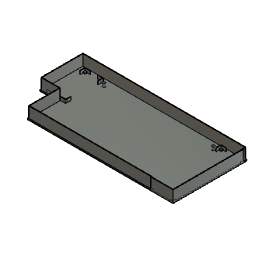
GeigerCounterBase v3 (Autodesk Fusion 360 design; units mm, degrees)
Autodesk Fusion 360 part; units mm, degrees
note: some values were not read from the file. Chosen so that the rebuilt part matches the saved one: which face or edge a step refers to; which pieces of a blend or face edit are solid.
(part 1 of 2)
sketch "Skizze1" plane through (0, 0, 0) normal (0, 1, 0) x (1, 0, 0)
  line L0 (0, 0) -> (133, 0)
  line L1 (133, 0) -> (133, -68.5)
  line L2 (133, -68.5) -> (0, -68.5)
  line L3 (0, -68.5) -> (0, 0)
  dimension "d1" = 133
  dimension "d2" = 68.5
  constraint horizontal L0
  constraint vertical L1
  constraint horizontal L2
  constraint vertical L3
  constraint coincident L0.start L3.end
  measures "d1" distance of L0.start L0.end
  measures "d2" distance of L0.start L2.end
extrude "Extrusion1" add sketch "Skizze1" along normal blind 1 makes body 1
sketch "Skizze2" plane through (0, 1, 0) normal (0, 1, 0) x (-1, 0, 0)
  line L0 (0, 68.5) -> (-133, 68.5)
  line L1 (-133, 68.5) -> (-133, 0)
  line L2 (-133, 0) -> (0, 0)
  line L3 (0, 0) -> (0, 68.5)
  circle A0 centre (-15, 10) radius 1.5
  dimension "d5" = 3
  measures "d5" diameter of A0
extrude "Extrusion2" add sketch "Skizze2" along normal blind 3 contours A0 bodies 1
pattern_linear "R-Anordnung1" count 2 spacing 10.15 along (1, 0, 0) of "Extrusion2"
delete_face "Fläche löschen1" 2 faces at (23.6519, 3, 9.9252) (25.4, 4, 10.4979) on bodies 1
delete_face "Fläche löschen2" 1 faces at (13.5019, 3, 9.9252) on bodies 1
sketch "Skizze3" plane through (0, 1, 0) normal (0, 1, 0) x (-1, 0, 0)
  line L0 (0, 68.5) -> (-133, 68.5)
  line L1 (-133, 68.5) -> (-133, 0)
  line L2 (-133, 0) -> (0, 0)
  line L3 (0, 0) -> (0, 68.5)
  circle A0 centre (-9.9603, 7.5483) radius 1.25
  dimension "d12" = 2.5
  measures "d12" diameter of A0
extrude "Extrusion3" add sketch "Skizze3" along normal blind 3 contours A0 bodies 1
pattern_linear "R-Anordnung2" count 2 spacing 101.5 along (1, 0, 0) of "Extrusion3"
pattern_linear "R-Anordnung3" count 2 spacing 56.5 along (0, 0, 1) of "Extrusion3"
pattern_linear "R-Anordnung4" count 2 spacing 101.5 along (1, 0, 0) of "R-Anordnung3"
sketch "Skizze4" plane through (0, 1, 0) normal (0, 1, 0) x (-1, 0, 0)
  circle A0 centre (-111.4603, 64.0483) radius 1.25
  circle A1 centre (-9.9603, 64.0483) radius 1.25
  circle A2 centre (-111.4603, 7.5483) radius 1.25
  circle A3 centre (-9.9603, 7.5483) radius 1.25
  line L0 (0, 68.5) -> (-133, 68.5)
  line L1 (-133, 68.5) -> (-133, 0)
  line L2 (-133, 0) -> (0, 0)
  line L3 (0, 0) -> (0, 68.5)
  line L4 (-133, 68.5) -> (-128, 68.5)
  line L5 (-128, 68.5) -> (-128, 68)
  line L6 (-128, 68) -> (-133, 68)
  line L7 (-133, 68) -> (-133, 68.5)
  dimension "d27" = 5
  constraint horizontal L4
  constraint vertical L5
  constraint horizontal L6
  constraint vertical L7
  constraint coincident L0.end L1.start
  measures "d27" distance of L0.end L4.end
extrude "Extrusion4" add sketch "Skizze4" along normal blind 3 contours L0 L1 L4 L5 L6 L7 bodies 1
sketch "Skizze5" plane through (0, 1, 0) normal (0, 1, 0) x (-1, 0, 0)
  line L0 (-128, 68.5) -> (-128, 68)
  line L1 (-128, 68) -> (-133, 68)
  line L2 (-133, 68) -> (-133, 0)
  line L3 (-133, 0) -> (0, 0)
  line L4 (0, 0) -> (0, 68.5)
  line L5 (0, 68.5) -> (-128, 68.5)
  circle A0 centre (-9.9603, 7.5483) radius 1.25
  circle A1 centre (-111.4603, 7.5483) radius 1.25
  circle A2 centre (-9.9603, 64.0483) radius 1.25
  circle A3 centre (-111.4603, 64.0483) radius 1.25
  line L6 (-133, 68) -> (-132.5, 68)
  line L7 (-132.5, 68) -> (-132.5, 63.5)
  line L8 (-132.5, 63.5) -> (-133, 63.5)
  line L9 (-133, 63.5) -> (-133, 68)
  dimension "d30" = 0.5
  dimension "d31" = 4.5
  constraint horizontal L6
  constraint vertical L7
  constraint horizontal L8
  constraint vertical L9
  constraint coincident L1.end L2.start
  measures "d30" distance of L1.end L6.end
  measures "d31" distance of L1.end L8.end
extrude "Extrusion5" add sketch "Skizze5" along normal blind 3 contours L1 L2 L6 L7 L8 L9 bodies 1
sketch "Skizze6" plane through (0, 1, 0) normal (0, 1, 0) x (-1, 0, 0)
  line L0 (-132.5, 63.5) -> (-133, 63.5)
  line L1 (-133, 63.5) -> (-133, 0)
  line L2 (-133, 0) -> (0, 0)
  line L3 (0, 0) -> (0, 68.5)
  line L4 (0, 68.5) -> (-128, 68.5)
  line L5 (-128, 68.5) -> (-128, 68)
  line L6 (-128, 68) -> (-132.5, 68)
  line L7 (-132.5, 68) -> (-132.5, 63.5)
  circle A0 centre (-9.9603, 7.5483) radius 1.25
  circle A1 centre (-111.4603, 7.5483) radius 1.25
  circle A2 centre (-9.9603, 64.0483) radius 1.25
  circle A3 centre (-111.4603, 64.0483) radius 1.25
  line L8 (-132.5, 68) -> (-130.5, 68)
  line L9 (-130.5, 68) -> (-130.5, 66)
  line L10 (-130.5, 66) -> (-132.5, 66)
  line L11 (-132.5, 66) -> (-132.5, 68)
  dimension "d34" = 2
  dimension "d35" = 2
  constraint horizontal L8
  constraint vertical L9
  constraint horizontal L10
  constraint vertical L11
  constraint coincident L6.end L7.start
  measures "d34" distance of L6.end L8.end
  measures "d35" distance of L6.end L10.end
extrude "Extrusion6" add sketch "Skizze6" along normal blind 1 contours L6 L7 L8 L9 L10 L11 bodies 1
sketch "Skizze7" plane through (0, 1, 0) normal (0, 1, 0) x (-1, 0, 0)
  line L0 (-130.5, 66) -> (-132.5, 66)
  line L1 (-132.5, 66) -> (-132.5, 63.5)
  line L2 (-132.5, 63.5) -> (-133, 63.5)
  line L3 (-133, 63.5) -> (-133, 0)
  line L4 (-133, 0) -> (0, 0)
  line L5 (0, 0) -> (0, 68.5)
  line L6 (0, 68.5) -> (-128, 68.5)
  line L7 (-128, 68.5) -> (-128, 68)
  line L8 (-128, 68) -> (-130.5, 68)
  line L9 (-130.5, 68) -> (-130.5, 66)
  circle A0 centre (-9.9603, 7.5483) radius 1.25
  circle A1 centre (-111.4603, 7.5483) radius 1.25
  circle A2 centre (-9.9603, 64.0483) radius 1.25
  circle A3 centre (-111.4603, 64.0483) radius 1.25
  line L10 (-135, 0) -> (-133, 0)
  line L11 (-133, 0) -> (-133, 68.5)
  line L12 (-133, 68.5) -> (-135, 68.5)
  line L13 (-135, 68.5) -> (-135, 0)
  dimension "d38" = 68.5
  constraint horizontal L10
  constraint vertical L11
  constraint horizontal L12
  constraint vertical L13
  measures "d38" distance of L10.start L12.end
extrude "Extrusion7" add sketch "Skizze7" against normal blind 1 contours L3 L10 L11 L12 L13 bodies 1
delete_face "Fläche löschen3" 1 faces at (133, 2, 66.8333) on bodies 1
sketch "Skizze8" plane through (0, 1, 0) normal (0, 1, 0) x (-1, 0, 0)
  circle A0 centre (-9.9603, 7.5483) radius 1.25
  circle A1 centre (-111.4603, 7.5483) radius 1.25
  circle A2 centre (-9.9603, 64.0483) radius 1.25
  circle A3 centre (-111.4603, 64.0483) radius 1.25
  line L0 (0, 68.5) -> (-135, 68.5)
  line L1 (-135, 68.5) -> (-135, 0)
  line L2 (-135, 0) -> (0, 0)
  line L3 (0, 0) -> (0, 68.5)
  line L4 (-135, 68.5) -> (-134.5, 68.5)
  line L5 (-134.5, 68.5) -> (-134.5, 63.5)
  line L6 (-134.5, 63.5) -> (-135, 63.5)
  line L7 (-135, 63.5) -> (-135, 68.5)
  dimension "d41" = 0.5
  dimension "d42" = 5
  constraint horizontal L4
  constraint vertical L5
  constraint horizontal L6
  constraint vertical L7
  constraint coincident L0.end L1.start
  measures "d41" distance of L0.end L4.end
  measures "d42" distance of L0.end L6.end
extrude "Extrusion8" add sketch "Skizze8" along normal blind 3 contours L0 L1 L4 L5 L6 L7 bodies 1
sketch "Skizze9" plane through (0, 1, 0) normal (0, 1, 0) x (-1, 0, 0)
  line L0 (-134.5, 68.5) -> (-134.5, 63.5)
  line L1 (-134.5, 63.5) -> (-135, 63.5)
  line L2 (-135, 63.5) -> (-135, 0)
  line L3 (-135, 0) -> (0, 0)
  line L4 (0, 0) -> (0, 68.5)
  line L5 (0, 68.5) -> (-134.5, 68.5)
  circle A0 centre (-111.4603, 64.0483) radius 1.25
  circle A1 centre (-9.9603, 64.0483) radius 1.25
  circle A2 centre (-111.4603, 7.5483) radius 1.25
  circle A3 centre (-9.9603, 7.5483) radius 1.25
  line L6 (-134.5, 68.5) -> (-130, 68.5)
  line L7 (-130, 68.5) -> (-130, 68)
  line L8 (-130, 68) -> (-134.5, 68)
  line L9 (-134.5, 68) -> (-134.5, 68.5)
  dimension "d45" = 4.5
  dimension "d46" = 0.5
  constraint horizontal L6
  constraint vertical L7
  constraint horizontal L8
  constraint vertical L9
  constraint coincident L0.start L5.end
  measures "d45" distance of L0.start L6.end
  measures "d46" distance of L0.start L8.end
extrude "Extrusion9" add sketch "Skizze9" along normal blind 3 contours L0 L5 L6 L7 L8 L9 bodies 1
sketch "Skizze10" plane through (0, 1, 0) normal (0, 1, 0) x (-1, 0, 0)
  circle A0 centre (-9.9603, 7.5483) radius 1.25
  circle A1 centre (-111.4603, 7.5483) radius 1.25
  circle A2 centre (-9.9603, 64.0483) radius 1.25
  circle A3 centre (-111.4603, 64.0483) radius 1.25
  line L0 (-130, 68.5) -> (-130, 68)
  line L1 (-130, 68) -> (-134.5, 68)
  line L2 (-134.5, 68) -> (-134.5, 63.5)
  line L3 (-134.5, 63.5) -> (-135, 63.5)
  line L4 (-135, 63.5) -> (-135, 0)
  line L5 (-135, 0) -> (0, 0)
  line L6 (0, 0) -> (0, 68.5)
  line L7 (0, 68.5) -> (-130, 68.5)
  line L8 (-114.094, 68.5) -> (-114.594, 68.5)
  line L9 (-114.594, 68.5) -> (-114.594, 63.5)
  line L10 (-114.594, 63.5) -> (-114.094, 63.5)
  line L11 (-114.094, 63.5) -> (-114.094, 68.5)
  dimension "d49" = 0.5
  dimension "d50" = 5
  constraint horizontal L8
  constraint vertical L9
  constraint horizontal L10
  constraint vertical L11
  constraint coincident L7 L8.start
  measures "d49" distance of L8.start L8.end
  measures "d50" distance of L8.start L10.end
extrude "Extrusion10" add sketch "Skizze10" along normal blind 3 contours L7 L8 L9 L10 L11 bodies 1
sketch "Skizze11" plane through (0, 1, 0) normal (0, 1, 0) x (-1, 0, 0)
  line L0 (-114.594, 63.5) -> (-114.594, 68.5)
  line L1 (-114.594, 68.5) -> (-130, 68.5)
  line L2 (-130, 68.5) -> (-130, 68)
  line L3 (-130, 68) -> (-134.5, 68)
  line L4 (-134.5, 68) -> (-134.5, 63.5)
  line L5 (-134.5, 63.5) -> (-135, 63.5)
  line L6 (-135, 63.5) -> (-135, 0)
  line L7 (-135, 0) -> (0, 0)
  line L8 (0, 0) -> (0, 68.5)
  line L9 (0, 68.5) -> (-114.094, 68.5)
  line L10 (-114.094, 68.5) -> (-114.094, 63.5)
  line L11 (-114.094, 63.5) -> (-114.594, 63.5)
  circle A0 centre (-9.9603, 7.5483) radius 1.25
  circle A1 centre (-111.4603, 7.5483) radius 1.25
  circle A2 centre (-9.9603, 64.0483) radius 1.25
  circle A3 centre (-111.4603, 64.0483) radius 1.25
  line L12 (-114.594, 68.5) -> (-119.094, 68.5)
  line L13 (-119.094, 68.5) -> (-119.094, 68)
  line L14 (-119.094, 68) -> (-114.594, 68)
  line L15 (-114.594, 68) -> (-114.594, 68.5)
  dimension "d53" = 4.5
  dimension "d54" = 0.5
  constraint horizontal L12
  constraint vertical L13
  constraint horizontal L14
  constraint vertical L15
  constraint coincident L0.end L1.start
  measures "d53" distance of L0.end L12.end
  measures "d54" distance of L0.end L14.end
extrude "Extrusion11" add sketch "Skizze11" along normal blind 3 contours L0 L1 L12 L13 L14 L15 bodies 1
sketch "Skizze12" plane through (0, 1, 0) normal (0, 1, 0) x (-1, 0, 0)
  circle A0 centre (-111.4603, 64.0483) radius 1.25
  circle A1 centre (-9.9603, 64.0483) radius 1.25
  circle A2 centre (-111.4603, 7.5483) radius 1.25
  circle A3 centre (-9.9603, 7.5483) radius 1.25
  line L0 (-114.594, 68) -> (-119.094, 68)
  line L1 (-119.094, 68) -> (-119.094, 68.5)
  line L2 (-119.094, 68.5) -> (-130, 68.5)
  line L3 (-130, 68.5) -> (-130, 68)
  line L4 (-130, 68) -> (-134.5, 68)
  line L5 (-134.5, 68) -> (-134.5, 63.5)
  line L6 (-134.5, 63.5) -> (-135, 63.5)
  line L7 (-135, 63.5) -> (-135, 0)
  line L8 (-135, 0) -> (0, 0)
  line L9 (0, 0) -> (0, 68.5)
  line L10 (0, 68.5) -> (-114.094, 68.5)
  line L11 (-114.094, 68.5) -> (-114.094, 63.5)
  line L12 (-114.094, 63.5) -> (-114.594, 63.5)
  line L13 (-114.594, 63.5) -> (-114.594, 68)
  line L14 (-135, 3) -> (-130, 3)
  line L15 (-130, 3) -> (-130, 3.5)
  line L16 (-130, 3.5) -> (-135, 3.5)
  line L17 (-135, 3.5) -> (-135, 3)
  dimension "d57" = 5
  dimension "d58" = 0.5
  constraint horizontal L14
  constraint vertical L15
  constraint horizontal L16
  constraint vertical L17
  constraint coincident L7 L14.start
  measures "d57" distance of L14.start L14.end
  measures "d58" distance of L14.start L16.end
extrude "Extrusion12" add sketch "Skizze12" along normal blind 3 contours L7 L14 L15 L16 L17 bodies 1
sketch "Skizze13" plane through (0, 1, 0) normal (0, 1, 0) x (-1, 0, 0)
  line L0 (-130, 3) -> (-135, 3)
  line L1 (-135, 3) -> (-135, 0)
  line L2 (-135, 0) -> (0, 0)
  line L3 (0, 0) -> (0, 68.5)
  line L4 (0, 68.5) -> (-114.094, 68.5)
  line L5 (-114.094, 68.5) -> (-114.094, 63.5)
  line L6 (-114.094, 63.5) -> (-114.594, 63.5)
  line L7 (-114.594, 63.5) -> (-114.594, 68)
  line L8 (-114.594, 68) -> (-119.094, 68)
  line L9 (-119.094, 68) -> (-119.094, 68.5)
  line L10 (-119.094, 68.5) -> (-130, 68.5)
  line L11 (-130, 68.5) -> (-130, 68)
  line L12 (-130, 68) -> (-134.5, 68)
  line L13 (-134.5, 68) -> (-134.5, 63.5)
  line L14 (-134.5, 63.5) -> (-135, 63.5)
  line L15 (-135, 63.5) -> (-135, 3.5)
  line L16 (-135, 3.5) -> (-130, 3.5)
  line L17 (-130, 3.5) -> (-130, 3)
  circle A0 centre (-111.4603, 64.0483) radius 1.25
  circle A1 centre (-9.9603, 64.0483) radius 1.25
  circle A2 centre (-111.4603, 7.5483) radius 1.25
  circle A3 centre (-9.9603, 7.5483) radius 1.25
  line L18 (-135, 3.5) -> (-134.5, 3.5)
  line L19 (-134.5, 3.5) -> (-134.5, 8.5)
  line L20 (-134.5, 8.5) -> (-135, 8.5)
  line L21 (-135, 8.5) -> (-135, 3.5)
  dimension "d61" = 0.5
  dimension "d62" = 5
  constraint horizontal L18
  constraint vertical L19
  constraint horizontal L20
  constraint vertical L21
  constraint coincident L15.end L16.start
  measures "d61" distance of L15.end L18.end
  measures "d62" distance of L15.end L20.end
extrude "Extrusion13" add sketch "Skizze13" along normal blind 3 contours L15 L16 L18 L19 L20 L21 bodies 1
sketch "Skizze14" plane through (0, 1, 0) normal (0, 1, 0) x (-1, 0, 0)
  circle A0 centre (-9.9603, 7.5483) radius 1.25
  circle A1 centre (-111.4603, 7.5483) radius 1.25
  circle A2 centre (-9.9603, 64.0483) radius 1.25
  circle A3 centre (-111.4603, 64.0483) radius 1.25
  line L0 (-135, 8.5) -> (-134.5, 8.5)
  line L1 (-134.5, 8.5) -> (-134.5, 3.5)
  line L2 (-134.5, 3.5) -> (-130, 3.5)
  line L3 (-130, 3.5) -> (-130, 3)
  line L4 (-130, 3) -> (-135, 3)
  line L5 (-135, 3) -> (-135, 0)
  line L6 (-135, 0) -> (0, 0)
  line L7 (0, 0) -> (0, 68.5)
  line L8 (0, 68.5) -> (-114.094, 68.5)
  line L9 (-114.094, 68.5) -> (-114.094, 63.5)
  line L10 (-114.094, 63.5) -> (-114.594, 63.5)
  line L11 (-114.594, 63.5) -> (-114.594, 68)
  line L12 (-114.594, 68) -> (-119.094, 68)
  line L13 (-119.094, 68) -> (-119.094, 68.5)
  line L14 (-119.094, 68.5) -> (-130, 68.5)
  line L15 (-130, 68.5) -> (-130, 68)
  line L16 (-130, 68) -> (-134.5, 68)
  line L17 (-134.5, 68) -> (-134.5, 63.5)
  line L18 (-134.5, 63.5) -> (-135, 63.5)
  line L19 (-135, 63.5) -> (-135, 8.5)
  line L20 (-114, 3) -> (-119, 3)
  line L21 (-119, 3) -> (-119, 3.5)
  line L22 (-119, 3.5) -> (-114, 3.5)
  line L23 (-114, 3.5) -> (-114, 3)
  dimension "d65" = 5
  constraint horizontal L20
  constraint vertical L21
  constraint horizontal L22
  constraint vertical L23
  measures "d65" distance of L20.start L20.end
extrude "Extrusion14" add sketch "Skizze14" along normal blind 3 contours L20 L21 L22 L23 bodies 1
sketch "Skizze15" plane through (0, 1, 0) normal (0, 1, 0) x (-1, 0, 0)
  line L0 (-114, 3.5) -> (-114, 3)
  line L1 (-114, 3) -> (-119, 3)
  line L2 (-119, 3) -> (-119, 3.5)
  line L3 (-119, 3.5) -> (-114, 3.5)
  circle A0 centre (-9.9603, 7.5483) radius 1.25
  circle A1 centre (-111.4603, 7.5483) radius 1.25
  circle A2 centre (-9.9603, 64.0483) radius 1.25
  circle A3 centre (-111.4603, 64.0483) radius 1.25
  line L4 (-135, 8.5) -> (-134.5, 8.5)
  line L5 (-134.5, 8.5) -> (-134.5, 3.5)
  line L6 (-134.5, 3.5) -> (-130, 3.5)
  line L7 (-130, 3.5) -> (-130, 3)
  line L8 (-130, 3) -> (-135, 3)
  line L9 (-135, 3) -> (-135, 0)
  line L10 (-135, 0) -> (0, 0)
  line L11 (0, 0) -> (0, 68.5)
  line L12 (0, 68.5) -> (-114.094, 68.5)
  line L13 (-114.094, 68.5) -> (-114.094, 63.5)
  line L14 (-114.094, 63.5) -> (-114.594, 63.5)
  line L15 (-114.594, 63.5) -> (-114.594, 68)
  line L16 (-114.594, 68) -> (-119.094, 68)
  line L17 (-119.094, 68) -> (-119.094, 68.5)
  line L18 (-119.094, 68.5) -> (-130, 68.5)
  line L19 (-130, 68.5) -> (-130, 68)
  line L20 (-130, 68) -> (-134.5, 68)
  line L21 (-134.5, 68) -> (-134.5, 63.5)
  line L22 (-134.5, 63.5) -> (-135, 63.5)
  line L23 (-135, 63.5) -> (-135, 8.5)
  line L24 (-114, 3.5) -> (-114.5, 3.5)
  line L25 (-114.5, 3.5) -> (-114.5, 8)
  line L26 (-114.5, 8) -> (-114, 8)
  line L27 (-114, 8) -> (-114, 3.5)
  dimension "d68" = 0.5
  dimension "d69" = 4.5
  constraint horizontal L24
  constraint vertical L25
  constraint horizontal L26
  constraint vertical L27
  constraint coincident L0.start L3.end
  measures "d68" distance of L0.start L24.end
  measures "d69" distance of L0.start L26.end
extrude "Extrusion15" add sketch "Skizze15" along normal blind 3 contours L3 L24 L25 L26 L27 bodies 1
sketch "Skizze16" plane through (0, 1, 0) normal (0, 1, 0) x (-1, 0, 0)
  line L0 (-135, 8.5) -> (-134.5, 8.5)
  line L1 (-134.5, 8.5) -> (-134.5, 3.5)
  line L2 (-134.5, 3.5) -> (-130, 3.5)
  line L3 (-130, 3.5) -> (-130, 3)
  line L4 (-130, 3) -> (-135, 3)
  line L5 (-135, 3) -> (-135, 0)
  line L6 (-135, 0) -> (0, 0)
  line L7 (0, 0) -> (0, 68.5)
  line L8 (0, 68.5) -> (-114.094, 68.5)
  line L9 (-114.094, 68.5) -> (-114.094, 63.5)
  line L10 (-114.094, 63.5) -> (-114.594, 63.5)
  line L11 (-114.594, 63.5) -> (-114.594, 68)
  line L12 (-114.594, 68) -> (-119.094, 68)
  line L13 (-119.094, 68) -> (-119.094, 68.5)
  line L14 (-119.094, 68.5) -> (-130, 68.5)
  line L15 (-130, 68.5) -> (-130, 68)
  line L16 (-130, 68) -> (-134.5, 68)
  line L17 (-134.5, 68) -> (-134.5, 63.5)
  line L18 (-134.5, 63.5) -> (-135, 63.5)
  line L19 (-135, 63.5) -> (-135, 8.5)
  circle A0 centre (-111.4603, 64.0483) radius 1.25
  circle A1 centre (-9.9603, 64.0483) radius 1.25
  circle A2 centre (-111.4603, 7.5483) radius 1.25
  circle A3 centre (-9.9603, 7.5483) radius 1.25
  line L20 (-114.5, 3.5) -> (-114.5, 8)
  line L21 (-114.5, 8) -> (-114, 8)
  line L22 (-114, 8) -> (-114, 3)
  line L23 (-114, 3) -> (-119, 3)
  line L24 (-119, 3) -> (-119, 3.5)
  line L25 (-119, 3.5) -> (-114.5, 3.5)
  line L26 (-134.5, 68) -> (-132.5, 68)
  line L27 (-132.5, 68) -> (-132.5, 66)
  line L28 (-132.5, 66) -> (-134.5, 66)
  line L29 (-134.5, 66) -> (-134.5, 68)
  dimension "d72" = 2
  dimension "d73" = 2
  constraint horizontal L26
  constraint vertical L27
  constraint horizontal L28
  constraint vertical L29
  constraint coincident L16.end L17.start
  measures "d72" distance of L16.end L26.end
  measures "d73" distance of L16.end L28.end
extrude "Extrusion16" add sketch "Skizze16" along normal blind 1 contours L16 L17 L26 L27 L28 L29 bodies 1
sketch "Skizze17" plane through (0, 1, 0) normal (0, 1, 0) x (-1, 0, 0)
  line L0 (-114.5, 3.5) -> (-114.5, 8)
  line L1 (-114.5, 8) -> (-114, 8)
  line L2 (-114, 8) -> (-114, 3)
  line L3 (-114, 3) -> (-119, 3)
  line L4 (-119, 3) -> (-119, 3.5)
  line L5 (-119, 3.5) -> (-114.5, 3.5)
  circle A0 centre (-9.9603, 7.5483) radius 1.25
  circle A1 centre (-111.4603, 7.5483) radius 1.25
  circle A2 centre (-9.9603, 64.0483) radius 1.25
  circle A3 centre (-111.4603, 64.0483) radius 1.25
  line L6 (-132.5, 68) -> (-132.5, 66)
  line L7 (-132.5, 66) -> (-134.5, 66)
  line L8 (-134.5, 66) -> (-134.5, 63.5)
  line L9 (-134.5, 63.5) -> (-135, 63.5)
  line L10 (-135, 63.5) -> (-135, 8.5)
  line L11 (-135, 8.5) -> (-134.5, 8.5)
  line L12 (-134.5, 8.5) -> (-134.5, 3.5)
  line L13 (-134.5, 3.5) -> (-130, 3.5)
  line L14 (-130, 3.5) -> (-130, 3)
  line L15 (-130, 3) -> (-135, 3)
  line L16 (-135, 3) -> (-135, 0)
  line L17 (-135, 0) -> (0, 0)
  line L18 (0, 0) -> (0, 68.5)
  line L19 (0, 68.5) -> (-114.094, 68.5)
  line L20 (-114.094, 68.5) -> (-114.094, 63.5)
  line L21 (-114.094, 63.5) -> (-114.594, 63.5)
  line L22 (-114.594, 63.5) -> (-114.594, 68)
  line L23 (-114.594, 68) -> (-119.094, 68)
  line L24 (-119.094, 68) -> (-119.094, 68.5)
  line L25 (-119.094, 68.5) -> (-130, 68.5)
  line L26 (-130, 68.5) -> (-130, 68)
  line L27 (-130, 68) -> (-132.5, 68)
  line L28 (-114.594, 68) -> (-116.594, 68)
  line L29 (-116.594, 68) -> (-116.594, 66)
  line L30 (-116.594, 66) -> (-114.594, 66)
  line L31 (-114.594, 66) -> (-114.594, 68)
  dimension "d76" = 2
  dimension "d77" = 2
  constraint horizontal L28
  constraint vertical L29
  constraint horizontal L30
  constraint vertical L31
  constraint coincident L22.end L23.start
  measures "d76" distance of L22.end L28.end
  measures "d77" distance of L22.end L30.end
extrude "Extrusion17" add sketch "Skizze17" along normal blind 1 contours L22 L23 L28 L29 L30 L31 bodies 1
sketch "Skizze18" plane through (0, 1, 0) normal (0, 1, 0) x (-1, 0, 0)
  line L0 (-116.594, 66) -> (-116.594, 68)
  line L1 (-116.594, 68) -> (-119.094, 68)
  line L2 (-119.094, 68) -> (-119.094, 68.5)
  line L3 (-119.094, 68.5) -> (-130, 68.5)
  line L4 (-130, 68.5) -> (-130, 68)
  line L5 (-130, 68) -> (-132.5, 68)
  line L6 (-132.5, 68) -> (-132.5, 66)
  line L7 (-132.5, 66) -> (-134.5, 66)
  line L8 (-134.5, 66) -> (-134.5, 63.5)
  line L9 (-134.5, 63.5) -> (-135, 63.5)
  line L10 (-135, 63.5) -> (-135, 8.5)
  line L11 (-135, 8.5) -> (-134.5, 8.5)
  line L12 (-134.5, 8.5) -> (-134.5, 3.5)
  line L13 (-134.5, 3.5) -> (-130, 3.5)
  line L14 (-130, 3.5) -> (-130, 3)
  line L15 (-130, 3) -> (-135, 3)
  line L16 (-135, 3) -> (-135, 0)
  line L17 (-135, 0) -> (0, 0)
  line L18 (0, 0) -> (0, 68.5)
  line L19 (0, 68.5) -> (-114.094, 68.5)
  line L20 (-114.094, 68.5) -> (-114.094, 63.5)
  line L21 (-114.094, 63.5) -> (-114.594, 63.5)
  line L22 (-114.594, 63.5) -> (-114.594, 66)
  line L23 (-114.594, 66) -> (-116.594, 66)
  line L24 (-114.5, 3.5) -> (-114.5, 8)
  line L25 (-114.5, 8) -> (-114, 8)
  line L26 (-114, 8) -> (-114, 3)
  line L27 (-114, 3) -> (-119, 3)
  line L28 (-119, 3) -> (-119, 3.5)
  line L29 (-119, 3.5) -> (-114.5, 3.5)
  circle A0 centre (-9.9603, 7.5483) radius 1.25
  circle A1 centre (-111.4603, 7.5483) radius 1.25
  circle A2 centre (-9.9603, 64.0483) radius 1.25
  circle A3 centre (-111.4603, 64.0483) radius 1.25
  line L30 (-134.5, 3.5) -> (-132.5, 3.5)
  line L31 (-132.5, 3.5) -> (-132.5, 5.5)
  line L32 (-132.5, 5.5) -> (-134.5, 5.5)
  line L33 (-134.5, 5.5) -> (-134.5, 3.5)
  dimension "d80" = 2
  dimension "d81" = 2
  constraint horizontal L30
  constraint vertical L31
  constraint horizontal L32
  constraint vertical L33
  constraint coincident L12.end L13.start
  measures "d80" distance of L12.end L30.end
  measures "d81" distance of L12.end L32.end
extrude "Extrusion18" add sketch "Skizze18" along normal blind 1 contours L12 L13 L30 L31 L32 L33 bodies 1
sketch "Skizze19" plane through (0, 1, 0) normal (0, 1, 0) x (-1, 0, 0)
  line L0 (-132.5, 5.5) -> (-132.5, 3.5)
  line L1 (-132.5, 3.5) -> (-130, 3.5)
  line L2 (-130, 3.5) -> (-130, 3)
  line L3 (-130, 3) -> (-135, 3)
  line L4 (-135, 3) -> (-135, 0)
  line L5 (-135, 0) -> (0, 0)
  line L6 (0, 0) -> (0, 68.5)
  line L7 (0, 68.5) -> (-114.094, 68.5)
  line L8 (-114.094, 68.5) -> (-114.094, 63.5)
  line L9 (-114.094, 63.5) -> (-114.594, 63.5)
  line L10 (-114.594, 63.5) -> (-114.594, 66)
  line L11 (-114.594, 66) -> (-116.594, 66)
  line L12 (-116.594, 66) -> (-116.594, 68)
  line L13 (-116.594, 68) -> (-119.094, 68)
  line L14 (-119.094, 68) -> (-119.094, 68.5)
  line L15 (-119.094, 68.5) -> (-130, 68.5)
  line L16 (-130, 68.5) -> (-130, 68)
  line L17 (-130, 68) -> (-132.5, 68)
  line L18 (-132.5, 68) -> (-132.5, 66)
  line L19 (-132.5, 66) -> (-134.5, 66)
  line L20 (-134.5, 66) -> (-134.5, 63.5)
  line L21 (-134.5, 63.5) -> (-135, 63.5)
  line L22 (-135, 63.5) -> (-135, 8.5)
  line L23 (-135, 8.5) -> (-134.5, 8.5)
  line L24 (-134.5, 8.5) -> (-134.5, 5.5)
  line L25 (-134.5, 5.5) -> (-132.5, 5.5)
  line L26 (-114.5, 3.5) -> (-114.5, 8)
  line L27 (-114.5, 8) -> (-114, 8)
  line L28 (-114, 8) -> (-114, 3)
  line L29 (-114, 3) -> (-119, 3)
  line L30 (-119, 3) -> (-119, 3.5)
  line L31 (-119, 3.5) -> (-114.5, 3.5)
  circle A0 centre (-9.9603, 7.5483) radius 1.25
  circle A1 centre (-111.4603, 7.5483) radius 1.25
  circle A2 centre (-9.9603, 64.0483) radius 1.25
  circle A3 centre (-111.4603, 64.0483) radius 1.25
  line L32 (-114.5, 3.5) -> (-116.5, 3.5)
  line L33 (-116.5, 3.5) -> (-116.5, 5.5)
  line L34 (-116.5, 5.5) -> (-114.5, 5.5)
  line L35 (-114.5, 5.5) -> (-114.5, 3.5)
  dimension "d84" = 2
  dimension "d85" = 2
  constraint horizontal L32
  constraint vertical L33
  constraint horizontal L34
  constraint vertical L35
  constraint coincident L26.start L31.end
  measures "d84" distance of L26.start L32.end
  measures "d85" distance of L26.start L34.end
extrude "Extrusion19" add sketch "Skizze19" along normal blind 1 contours L26 L31 L32 L33 L34 L35 bodies 1
sketch "Skizze20" plane through (0, 0, 0) normal (0, 1, 0) x (1, 0, 0)
  line L0 (0, 0) -> (-17, 0)
  line L1 (-17, 0) -> (-17, -40)
  line L2 (-17, -40) -> (0, -40)
  line L3 (0, -40) -> (0, 0)
  dimension "d88" = 17
  dimension "d89" = 40
  constraint horizontal L0
  constraint vertical L1
  constraint horizontal L2
  constraint vertical L3
  constraint coincident L0.start L3.end
  measures "d88" distance of L0.start L0.end
  measures "d89" distance of L0.start L2.end
extrude "Extrusion20" add sketch "Skizze20" along normal blind 1 bodies 1
sketch "Skizze21" plane through (0, 1, 0) normal (0, 1, 0) x (-1, 0, 0)
  circle A0 centre (-111.4603, 64.0483) radius 1.25
  circle A1 centre (-9.9603, 64.0483) radius 1.25
  circle A2 centre (-111.4603, 7.5483) radius 1.25
  circle A3 centre (-9.9603, 7.5483) radius 1.25
  line L0 (-116.5, 3.5) -> (-116.5, 5.5)
  line L1 (-116.5, 5.5) -> (-114.5, 5.5)
  line L2 (-114.5, 5.5) -> (-114.5, 8)
  line L3 (-114.5, 8) -> (-114, 8)
  line L4 (-114, 8) -> (-114, 3)
  line L5 (-114, 3) -> (-119, 3)
  line L6 (-119, 3) -> (-119, 3.5)
  line L7 (-119, 3.5) -> (-116.5, 3.5)
  line L8 (-132.5, 5.5) -> (-132.5, 3.5)
  line L9 (-132.5, 3.5) -> (-130, 3.5)
  line L10 (-130, 3.5) -> (-130, 3)
  line L11 (-130, 3) -> (-135, 3)
  line L12 (-135, 3) -> (-135, 0)
  line L13 (-135, 0) -> (17, 0)
  line L14 (17, 0) -> (17, 40)
  line L15 (17, 40) -> (0, 40)
  line L16 (0, 40) -> (0, 68.5)
  line L17 (0, 68.5) -> (-114.094, 68.5)
  line L18 (-114.094, 68.5) -> (-114.094, 63.5)
  line L19 (-114.094, 63.5) -> (-114.594, 63.5)
  line L20 (-114.594, 63.5) -> (-114.594, 66)
  line L21 (-114.594, 66) -> (-116.594, 66)
  line L22 (-116.594, 66) -> (-116.594, 68)
  line L23 (-116.594, 68) -> (-119.094, 68)
  line L24 (-119.094, 68) -> (-119.094, 68.5)
  line L25 (-119.094, 68.5) -> (-130, 68.5)
  line L26 (-130, 68.5) -> (-130, 68)
  line L27 (-130, 68) -> (-132.5, 68)
  line L28 (-132.5, 68) -> (-132.5, 66)
  line L29 (-132.5, 66) -> (-134.5, 66)
  line L30 (-134.5, 66) -> (-134.5, 63.5)
  line L31 (-134.5, 63.5) -> (-135, 63.5)
  line L32 (-135, 63.5) -> (-135, 8.5)
  line L33 (-135, 8.5) -> (-134.5, 8.5)
  line L34 (-134.5, 8.5) -> (-134.5, 5.5)
  line L35 (-134.5, 5.5) -> (-132.5, 5.5)
  line L36 (-6, 4) -> (-1, 4)
  line L37 (-1, 4) -> (-1, 4.5)
  line L38 (-1, 4.5) -> (-6, 4.5)
  line L39 (-6, 4.5) -> (-6, 4)
  dimension "d92" = 5
  dimension "d93" = 0.5
  constraint horizontal L36
  constraint vertical L37
  constraint horizontal L38
  constraint vertical L39
  measures "d92" distance of L36.start L36.end
  measures "d93" distance of L36.start L38.end
extrude "Extrusion21" add sketch "Skizze21" along normal blind 3 contours L36 L37 L38 L39 bodies 1
sketch "Skizze22" plane through (0, 1, 0) normal (0, 1, 0) x (-1, 0, 0)
  line L0 (-6, 4.5) -> (-1, 4.5)
  line L1 (-1, 4.5) -> (-1, 4)
  line L2 (-1, 4) -> (-6, 4)
  line L3 (-6, 4) -> (-6, 4.5)
  circle A0 centre (-111.4603, 64.0483) radius 1.25
  circle A1 centre (-9.9603, 64.0483) radius 1.25
  circle A2 centre (-111.4603, 7.5483) radius 1.25
  circle A3 centre (-9.9603, 7.5483) radius 1.25
  line L4 (-116.5, 3.5) -> (-116.5, 5.5)
  line L5 (-116.5, 5.5) -> (-114.5, 5.5)
  line L6 (-114.5, 5.5) -> (-114.5, 8)
  line L7 (-114.5, 8) -> (-114, 8)
  line L8 (-114, 8) -> (-114, 3)
  line L9 (-114, 3) -> (-119, 3)
  line L10 (-119, 3) -> (-119, 3.5)
  line L11 (-119, 3.5) -> (-116.5, 3.5)
  line L12 (-132.5, 5.5) -> (-132.5, 3.5)
  line L13 (-132.5, 3.5) -> (-130, 3.5)
  line L14 (-130, 3.5) -> (-130, 3)
  line L15 (-130, 3) -> (-135, 3)
  line L16 (-135, 3) -> (-135, 0)
  line L17 (-135, 0) -> (17, 0)
  line L18 (17, 0) -> (17, 40)
  line L19 (17, 40) -> (0, 40)
  line L20 (0, 40) -> (0, 68.5)
  line L21 (0, 68.5) -> (-114.094, 68.5)
  line L22 (-114.094, 68.5) -> (-114.094, 63.5)
  line L23 (-114.094, 63.5) -> (-114.594, 63.5)
  line L24 (-114.594, 63.5) -> (-114.594, 66)
  line L25 (-114.594, 66) -> (-116.594, 66)
  line L26 (-116.594, 66) -> (-116.594, 68)
  line L27 (-116.594, 68) -> (-119.094, 68)
  line L28 (-119.094, 68) -> (-119.094, 68.5)
  line L29 (-119.094, 68.5) -> (-130, 68.5)
  line L30 (-130, 68.5) -> (-130, 68)
  line L31 (-130, 68) -> (-132.5, 68)
  line L32 (-132.5, 68) -> (-132.5, 66)
  line L33 (-132.5, 66) -> (-134.5, 66)
  line L34 (-134.5, 66) -> (-134.5, 63.5)
  line L35 (-134.5, 63.5) -> (-135, 63.5)
  line L36 (-135, 63.5) -> (-135, 8.5)
  line L37 (-135, 8.5) -> (-134.5, 8.5)
  line L38 (-134.5, 8.5) -> (-134.5, 5.5)
  line L39 (-134.5, 5.5) -> (-132.5, 5.5)
  line L40 (-6, 4.5) -> (-5.5, 4.5)
  line L41 (-5.5, 4.5) -> (-5.5, 8.4372)
  line L42 (-5.5, 8.4372) -> (-6, 8.4372)
  line L43 (-6, 8.4372) -> (-6, 4.5)
  dimension "d96" = 0.5
  dimension "d97" = 3.9372
  constraint horizontal L40
  constraint vertical L41
  constraint horizontal L42
  constraint vertical L43
  constraint coincident L0.start L3.end
  measures "d96" distance of L0.start L40.end
  measures "d97" distance of L0.start L42.end
extrude "Extrusion22" add sketch "Skizze22" along normal blind 3 contours L0 L40 L41 L42 L43 bodies 1
sketch "Skizze23" plane through (0, 1, 0) normal (0, 1, 0) x (-1, 0, 0)
  line L0 (-5.5, 8.4372) -> (-5.5, 4.5)
  line L1 (-5.5, 4.5) -> (-1, 4.5)
  line L2 (-1, 4.5) -> (-1, 4)
  line L3 (-1, 4) -> (-6, 4)
  line L4 (-6, 4) -> (-6, 8.4372)
  line L5 (-6, 8.4372) -> (-5.5, 8.4372)
  circle A0 centre (-111.4603, 64.0483) radius 1.25
  circle A1 centre (-9.9603, 64.0483) radius 1.25
  circle A2 centre (-111.4603, 7.5483) radius 1.25
  circle A3 centre (-9.9603, 7.5483) radius 1.25
  line L6 (-116.5, 3.5) -> (-116.5, 5.5)
  line L7 (-116.5, 5.5) -> (-114.5, 5.5)
  line L8 (-114.5, 5.5) -> (-114.5, 8)
  line L9 (-114.5, 8) -> (-114, 8)
  line L10 (-114, 8) -> (-114, 3)
  line L11 (-114, 3) -> (-119, 3)
  line L12 (-119, 3) -> (-119, 3.5)
  line L13 (-119, 3.5) -> (-116.5, 3.5)
  line L14 (-132.5, 5.5) -> (-132.5, 3.5)
  line L15 (-132.5, 3.5) -> (-130, 3.5)
  line L16 (-130, 3.5) -> (-130, 3)
  line L17 (-130, 3) -> (-135, 3)
  line L18 (-135, 3) -> (-135, 0)
  line L19 (-135, 0) -> (17, 0)
  line L20 (17, 0) -> (17, 40)
  line L21 (17, 40) -> (0, 40)
  line L22 (0, 40) -> (0, 68.5)
  line L23 (0, 68.5) -> (-114.094, 68.5)
  line L24 (-114.094, 68.5) -> (-114.094, 63.5)
  line L25 (-114.094, 63.5) -> (-114.594, 63.5)
  line L26 (-114.594, 63.5) -> (-114.594, 66)
  line L27 (-114.594, 66) -> (-116.594, 66)
  line L28 (-116.594, 66) -> (-116.594, 68)
  line L29 (-116.594, 68) -> (-119.094, 68)
  line L30 (-119.094, 68) -> (-119.094, 68.5)
  line L31 (-119.094, 68.5) -> (-130, 68.5)
  line L32 (-130, 68.5) -> (-130, 68)
  line L33 (-130, 68) -> (-132.5, 68)
  line L34 (-132.5, 68) -> (-132.5, 66)
  line L35 (-132.5, 66) -> (-134.5, 66)
  line L36 (-134.5, 66) -> (-134.5, 63.5)
  line L37 (-134.5, 63.5) -> (-135, 63.5)
  line L38 (-135, 63.5) -> (-135, 8.5)
  line L39 (-135, 8.5) -> (-134.5, 8.5)
  line L40 (-134.5, 8.5) -> (-134.5, 5.5)
  line L41 (-134.5, 5.5) -> (-132.5, 5.5)
  line L42 (11, 4) -> (6, 4)
  line L43 (6, 4) -> (6, 4.5)
  line L44 (6, 4.5) -> (11, 4.5)
  line L45 (11, 4.5) -> (11, 4)
  dimension "d100" = 5
  dimension "d101" = 0.5
  constraint horizontal L42
  constraint vertical L43
  constraint horizontal L44
  constraint vertical L45
  measures "d100" distance of L42.start L42.end
  measures "d101" distance of L42.start L44.end
extrude "Extrusion23" add sketch "Skizze23" along normal blind 3 contours L42 L43 L44 L45 bodies 1
sketch "Skizze24" plane through (0, 1, 0) normal (0, 1, 0) x (-1, 0, 0)
  line L0 (11, 4.5) -> (11, 4)
  line L1 (11, 4) -> (6, 4)
  line L2 (6, 4) -> (6, 4.5)
  line L3 (6, 4.5) -> (11, 4.5)
  line L4 (-5.5, 8.4372) -> (-5.5, 4.5)
  line L5 (-5.5, 4.5) -> (-1, 4.5)
  line L6 (-1, 4.5) -> (-1, 4)
  line L7 (-1, 4) -> (-6, 4)
  line L8 (-6, 4) -> (-6, 8.4372)
  line L9 (-6, 8.4372) -> (-5.5, 8.4372)
  circle A0 centre (-111.4603, 64.0483) radius 1.25
  circle A1 centre (-9.9603, 64.0483) radius 1.25
  circle A2 centre (-111.4603, 7.5483) radius 1.25
  circle A3 centre (-9.9603, 7.5483) radius 1.25
  line L10 (-116.5, 3.5) -> (-116.5, 5.5)
  line L11 (-116.5, 5.5) -> (-114.5, 5.5)
  line L12 (-114.5, 5.5) -> (-114.5, 8)
  line L13 (-114.5, 8) -> (-114, 8)
  line L14 (-114, 8) -> (-114, 3)
  line L15 (-114, 3) -> (-119, 3)
  line L16 (-119, 3) -> (-119, 3.5)
  line L17 (-119, 3.5) -> (-116.5, 3.5)
  line L18 (-132.5, 5.5) -> (-132.5, 3.5)
  line L19 (-132.5, 3.5) -> (-130, 3.5)
  line L20 (-130, 3.5) -> (-130, 3)
  line L21 (-130, 3) -> (-135, 3)
  line L22 (-135, 3) -> (-135, 0)
  line L23 (-135, 0) -> (17, 0)
  line L24 (17, 0) -> (17, 40)
  line L25 (17, 40) -> (0, 40)
  line L26 (0, 40) -> (0, 68.5)
  line L27 (0, 68.5) -> (-114.094, 68.5)
  line L28 (-114.094, 68.5) -> (-114.094, 63.5)
  line L29 (-114.094, 63.5) -> (-114.594, 63.5)
  line L30 (-114.594, 63.5) -> (-114.594, 66)
  line L31 (-114.594, 66) -> (-116.594, 66)
  line L32 (-116.594, 66) -> (-116.594, 68)
  line L33 (-116.594, 68) -> (-119.094, 68)
  line L34 (-119.094, 68) -> (-119.094, 68.5)
  line L35 (-119.094, 68.5) -> (-130, 68.5)
  line L36 (-130, 68.5) -> (-130, 68)
  line L37 (-130, 68) -> (-132.5, 68)
  line L38 (-132.5, 68) -> (-132.5, 66)
  line L39 (-132.5, 66) -> (-134.5, 66)
  line L40 (-134.5, 66) -> (-134.5, 63.5)
  line L41 (-134.5, 63.5) -> (-135, 63.5)
  line L42 (-135, 63.5) -> (-135, 8.5)
  line L43 (-135, 8.5) -> (-134.5, 8.5)
  line L44 (-134.5, 8.5) -> (-134.5, 5.5)
  line L45 (-134.5, 5.5) -> (-132.5, 5.5)
  line L46 (11, 4.5) -> (10.5, 4.5)
  line L47 (10.5, 4.5) -> (10.5, 9)
  line L48 (10.5, 9) -> (11, 9)
  line L49 (11, 9) -> (11, 4.5)
  dimension "d104" = 0.5
  dimension "d105" = 4.5
  constraint horizontal L46
  constraint vertical L47
  constraint horizontal L48
  constraint vertical L49
  constraint coincident L0.start L3.end
  measures "d104" distance of L0.start L46.end
  measures "d105" distance of L0.start L48.end
extrude "Extrusion24" add sketch "Skizze24" along normal blind 3 contours L3 L46 L47 L48 L49 bodies 1
sketch "Skizze25" plane through (0, 4, 0) normal (0, 1, 0) x (-1, 0, 0)
  line L0 (-6, 8.4372) -> (-6, 4)
  line L1 (-6, 4) -> (-1, 4)
  line L2 (-1, 4) -> (-1, 4.5)
  line L3 (-1, 4.5) -> (-5.5, 4.5)
  line L4 (-5.5, 4.5) -> (-5.5, 8.4372)
  line L5 (-5.5, 8.4372) -> (-6, 8.4372)
  line L6 (-6, 8.4372) -> (-5.5, 8.4372)
  line L7 (-5.5, 8.4372) -> (-5.5, 8.9372)
  line L8 (-5.5, 8.9372) -> (-6, 8.9372)
  line L9 (-6, 8.9372) -> (-6, 8.4372)
  dimension "d108" = 0.5
  dimension "d109" = 0.5
  constraint horizontal L6
  constraint vertical L7
  constraint horizontal L8
  constraint vertical L9
  constraint coincident L0.start L5.end
  measures "d108" distance of L0.start L4.end
  measures "d109" distance of L0.start L8.end
extrude "Extrusion25" add sketch "Skizze25" against normal blind 3 contours L5 L6 L7 L8 L9 bodies 1
sketch "Skizze26" plane through (0, 1, 0) normal (0, 1, 0) x (-1, 0, 0)
  line L0 (-5.5, 8.9372) -> (-5.5, 4.5)
  line L1 (-5.5, 4.5) -> (-1, 4.5)
  line L2 (-1, 4.5) -> (-1, 4)
  line L3 (-1, 4) -> (-6, 4)
  line L4 (-6, 4) -> (-6, 8.9372)
  line L5 (-6, 8.9372) -> (-5.5, 8.9372)
  line L6 (-132.5, 5.5) -> (-132.5, 3.5)
  line L7 (-132.5, 3.5) -> (-130, 3.5)
  line L8 (-130, 3.5) -> (-130, 3)
  line L9 (-130, 3) -> (-135, 3)
  line L10 (-135, 3) -> (-135, 0)
  line L11 (-135, 0) -> (17, 0)
  line L12 (17, 0) -> (17, 40)
  line L13 (17, 40) -> (0, 40)
  line L14 (0, 40) -> (0, 68.5)
  line L15 (0, 68.5) -> (-114.094, 68.5)
  line L16 (-114.094, 68.5) -> (-114.094, 63.5)
  line L17 (-114.094, 63.5) -> (-114.594, 63.5)
  line L18 (-114.594, 63.5) -> (-114.594, 66)
  line L19 (-114.594, 66) -> (-116.594, 66)
  line L20 (-116.594, 66) -> (-116.594, 68)
  line L21 (-116.594, 68) -> (-119.094, 68)
  line L22 (-119.094, 68) -> (-119.094, 68.5)
  line L23 (-119.094, 68.5) -> (-130, 68.5)
  line L24 (-130, 68.5) -> (-130, 68)
  line L25 (-130, 68) -> (-132.5, 68)
  line L26 (-132.5, 68) -> (-132.5, 66)
  line L27 (-132.5, 66) -> (-134.5, 66)
  line L28 (-134.5, 66) -> (-134.5, 63.5)
  line L29 (-134.5, 63.5) -> (-135, 63.5)
  line L30 (-135, 63.5) -> (-135, 8.5)
  line L31 (-135, 8.5) -> (-134.5, 8.5)
  line L32 (-134.5, 8.5) -> (-134.5, 5.5)
  line L33 (-134.5, 5.5) -> (-132.5, 5.5)
  line L34 (-116.5, 3.5) -> (-116.5, 5.5)
  line L35 (-116.5, 5.5) -> (-114.5, 5.5)
  line L36 (-114.5, 5.5) -> (-114.5, 8)
  line L37 (-114.5, 8) -> (-114, 8)
  line L38 (-114, 8) -> (-114, 3)
  line L39 (-114, 3) -> (-119, 3)
  line L40 (-119, 3) -> (-119, 3.5)
  line L41 (-119, 3.5) -> (-116.5, 3.5)
  circle A0 centre (-9.9603, 7.5483) radius 1.25
  circle A1 centre (-111.4603, 7.5483) radius 1.25
  circle A2 centre (-9.9603, 64.0483) radius 1.25
  circle A3 centre (-111.4603, 64.0483) radius 1.25
  line L42 (10.5, 4.5) -> (10.5, 9)
  line L43 (10.5, 9) -> (11, 9)
  line L44 (11, 9) -> (11, 4)
  line L45 (11, 4) -> (6, 4)
  line L46 (6, 4) -> (6, 4.5)
  line L47 (6, 4.5) -> (10.5, 4.5)
  line L48 (11, 39) -> (6, 39)
  line L49 (6, 39) -> (6, 38.5)
  line L50 (6, 38.5) -> (11, 38.5)
  line L51 (11, 38.5) -> (11, 39)
  dimension "d112" = 5
  dimension "d113" = 0.5
  constraint horizontal L48
  constraint vertical L49
  constraint horizontal L50
  constraint vertical L51
  measures "d112" distance of L48.start L48.end
  measures "d113" distance of L48.start L50.end
extrude "Extrusion26" add sketch "Skizze26" along normal blind 3 contours L48 L49 L50 L51 bodies 1
sketch "Skizze27" plane through (0, 1, 0) normal (0, 1, 0) x (-1, 0, 0)
  line L0 (11, 38.5) -> (6, 38.5)
  line L1 (6, 38.5) -> (6, 39)
  line L2 (6, 39) -> (11, 39)
  line L3 (11, 39) -> (11, 38.5)
  line L4 (-5.5, 8.9372) -> (-5.5, 4.5)
  line L5 (-5.5, 4.5) -> (-1, 4.5)
  line L6 (-1, 4.5) -> (-1, 4)
  line L7 (-1, 4) -> (-6, 4)
  line L8 (-6, 4) -> (-6, 8.9372)
  line L9 (-6, 8.9372) -> (-5.5, 8.9372)
  line L10 (-132.5, 5.5) -> (-132.5, 3.5)
  line L11 (-132.5, 3.5) -> (-130, 3.5)
  line L12 (-130, 3.5) -> (-130, 3)
  line L13 (-130, 3) -> (-135, 3)
  line L14 (-135, 3) -> (-135, 0)
  line L15 (-135, 0) -> (17, 0)
  line L16 (17, 0) -> (17, 40)
  line L17 (17, 40) -> (0, 40)
  line L18 (0, 40) -> (0, 68.5)
  line L19 (0, 68.5) -> (-114.094, 68.5)
  line L20 (-114.094, 68.5) -> (-114.094, 63.5)
  line L21 (-114.094, 63.5) -> (-114.594, 63.5)
  line L22 (-114.594, 63.5) -> (-114.594, 66)
  line L23 (-114.594, 66) -> (-116.594, 66)
  line L24 (-116.594, 66) -> (-116.594, 68)
  line L25 (-116.594, 68) -> (-119.094, 68)
  line L26 (-119.094, 68) -> (-119.094, 68.5)
  line L27 (-119.094, 68.5) -> (-130, 68.5)
  line L28 (-130, 68.5) -> (-130, 68)
  line L29 (-130, 68) -> (-132.5, 68)
  line L30 (-132.5, 68) -> (-132.5, 66)
  line L31 (-132.5, 66) -> (-134.5, 66)
  line L32 (-134.5, 66) -> (-134.5, 63.5)
  line L33 (-134.5, 63.5) -> (-135, 63.5)
  line L34 (-135, 63.5) -> (-135, 8.5)
  line L35 (-135, 8.5) -> (-134.5, 8.5)
  line L36 (-134.5, 8.5) -> (-134.5, 5.5)
  line L37 (-134.5, 5.5) -> (-132.5, 5.5)
  line L38 (-116.5, 3.5) -> (-116.5, 5.5)
  line L39 (-116.5, 5.5) -> (-114.5, 5.5)
  line L40 (-114.5, 5.5) -> (-114.5, 8)
  line L41 (-114.5, 8) -> (-114, 8)
  line L42 (-114, 8) -> (-114, 3)
  line L43 (-114, 3) -> (-119, 3)
  line L44 (-119, 3) -> (-119, 3.5)
  line L45 (-119, 3.5) -> (-116.5, 3.5)
  circle A0 centre (-9.9603, 7.5483) radius 1.25
  circle A1 centre (-111.4603, 7.5483) radius 1.25
  circle A2 centre (-9.9603, 64.0483) radius 1.25
  circle A3 centre (-111.4603, 64.0483) radius 1.25
  line L46 (10.5, 4.5) -> (10.5, 9)
  line L47 (10.5, 9) -> (11, 9)
  line L48 (11, 9) -> (11, 4)
  line L49 (11, 4) -> (6, 4)
  line L50 (6, 4) -> (6, 4.5)
  line L51 (6, 4.5) -> (10.5, 4.5)
  line L52 (11, 38.5) -> (10.5, 38.5)
  line L53 (10.5, 38.5) -> (10.5, 34)
  line L54 (10.5, 34) -> (11, 34)
  line L55 (11, 34) -> (11, 38.5)
  dimension "d116" = 0.5
  dimension "d117" = 4.5
  constraint horizontal L52
  constraint vertical L53
  constraint horizontal L54
  constraint vertical L55
  constraint coincident L0.start L3.end
  measures "d116" distance of L0.start L52.end
  measures "d117" distance of L0.start L54.end
extrude "Extrusion27" add sketch "Skizze27" along normal blind 3 contours L0 L52 L53 L54 L55 bodies 1
sketch "Skizze28" plane through (0, 1, 0) normal (0, 1, 0) x (-1, 0, 0)
  line L0 (10.5, 34) -> (10.5, 38.5)
  line L1 (10.5, 38.5) -> (6, 38.5)
  line L2 (6, 38.5) -> (6, 39)
  line L3 (6, 39) -> (11, 39)
  line L4 (11, 39) -> (11, 34)
  line L5 (11, 34) -> (10.5, 34)
  line L6 (-5.5, 8.9372) -> (-5.5, 4.5)
  line L7 (-5.5, 4.5) -> (-1, 4.5)
  line L8 (-1, 4.5) -> (-1, 4)
  line L9 (-1, 4) -> (-6, 4)
  line L10 (-6, 4) -> (-6, 8.9372)
  line L11 (-6, 8.9372) -> (-5.5, 8.9372)
  line L12 (-132.5, 5.5) -> (-132.5, 3.5)
  line L13 (-132.5, 3.5) -> (-130, 3.5)
  line L14 (-130, 3.5) -> (-130, 3)
  line L15 (-130, 3) -> (-135, 3)
  line L16 (-135, 3) -> (-135, 0)
  line L17 (-135, 0) -> (17, 0)
  line L18 (17, 0) -> (17, 40)
  line L19 (17, 40) -> (0, 40)
  line L20 (0, 40) -> (0, 68.5)
  line L21 (0, 68.5) -> (-114.094, 68.5)
  line L22 (-114.094, 68.5) -> (-114.094, 63.5)
  line L23 (-114.094, 63.5) -> (-114.594, 63.5)
  line L24 (-114.594, 63.5) -> (-114.594, 66)
  line L25 (-114.594, 66) -> (-116.594, 66)
  line L26 (-116.594, 66) -> (-116.594, 68)
  line L27 (-116.594, 68) -> (-119.094, 68)
  line L28 (-119.094, 68) -> (-119.094, 68.5)
  line L29 (-119.094, 68.5) -> (-130, 68.5)
  line L30 (-130, 68.5) -> (-130, 68)
  line L31 (-130, 68) -> (-132.5, 68)
  line L32 (-132.5, 68) -> (-132.5, 66)
  line L33 (-132.5, 66) -> (-134.5, 66)
  line L34 (-134.5, 66) -> (-134.5, 63.5)
  line L35 (-134.5, 63.5) -> (-135, 63.5)
  line L36 (-135, 63.5) -> (-135, 8.5)
  line L37 (-135, 8.5) -> (-134.5, 8.5)
  line L38 (-134.5, 8.5) -> (-134.5, 5.5)
  line L39 (-134.5, 5.5) -> (-132.5, 5.5)
  line L40 (-116.5, 3.5) -> (-116.5, 5.5)
  line L41 (-116.5, 5.5) -> (-114.5, 5.5)
  line L42 (-114.5, 5.5) -> (-114.5, 8)
  line L43 (-114.5, 8) -> (-114, 8)
  line L44 (-114, 8) -> (-114, 3)
  line L45 (-114, 3) -> (-119, 3)
  line L46 (-119, 3) -> (-119, 3.5)
  line L47 (-119, 3.5) -> (-116.5, 3.5)
  circle A0 centre (-9.9603, 7.5483) radius 1.25
  circle A1 centre (-111.4603, 7.5483) radius 1.25
  circle A2 centre (-9.9603, 64.0483) radius 1.25
  circle A3 centre (-111.4603, 64.0483) radius 1.25
  line L48 (10.5, 4.5) -> (10.5, 9)
  line L49 (10.5, 9) -> (11, 9)
  line L50 (11, 9) -> (11, 4)
  line L51 (11, 4) -> (6, 4)
  line L52 (6, 4) -> (6, 4.5)
  line L53 (6, 4.5) -> (10.5, 4.5)
  line L54 (-6, 39) -> (-1, 39)
  line L55 (-1, 39) -> (-1, 38.5)
  line L56 (-1, 38.5) -> (-6, 38.5)
  line L57 (-6, 38.5) -> (-6, 39)
  dimension "d120" = 5
  dimension "d121" = 0.5
  constraint horizontal L54
  constraint vertical L55
  constraint horizontal L56
  constraint vertical L57
  measures "d120" distance of L54.start L54.end
  measures "d121" distance of L54.start L56.end
extrude "Extrusion28" add sketch "Skizze28" along normal blind 3 contours L54 L55 L56 L57 bodies 1
sketch "Skizze29" plane through (0, 1, 0) normal (0, 1, 0) x (-1, 0, 0)
  line L0 (-6, 38.5) -> (-6, 39)
  line L1 (-6, 39) -> (-1, 39)
  line L2 (-1, 39) -> (-1, 38.5)
  line L3 (-1, 38.5) -> (-6, 38.5)
  line L4 (10.5, 34) -> (10.5, 38.5)
  line L5 (10.5, 38.5) -> (6, 38.5)
  line L6 (6, 38.5) -> (6, 39)
  line L7 (6, 39) -> (11, 39)
  line L8 (11, 39) -> (11, 34)
  line L9 (11, 34) -> (10.5, 34)
  line L10 (-5.5, 8.9372) -> (-5.5, 4.5)
  line L11 (-5.5, 4.5) -> (-1, 4.5)
  line L12 (-1, 4.5) -> (-1, 4)
  line L13 (-1, 4) -> (-6, 4)
  line L14 (-6, 4) -> (-6, 8.9372)
  line L15 (-6, 8.9372) -> (-5.5, 8.9372)
  line L16 (-132.5, 5.5) -> (-132.5, 3.5)
  line L17 (-132.5, 3.5) -> (-130, 3.5)
  line L18 (-130, 3.5) -> (-130, 3)
  line L19 (-130, 3) -> (-135, 3)
  line L20 (-135, 3) -> (-135, 0)
  line L21 (-135, 0) -> (17, 0)
  line L22 (17, 0) -> (17, 40)
  line L23 (17, 40) -> (0, 40)
  line L24 (0, 40) -> (0, 68.5)
  line L25 (0, 68.5) -> (-114.094, 68.5)
  line L26 (-114.094, 68.5) -> (-114.094, 63.5)
  line L27 (-114.094, 63.5) -> (-114.594, 63.5)
  line L28 (-114.594, 63.5) -> (-114.594, 66)
  line L29 (-114.594, 66) -> (-116.594, 66)
  line L30 (-116.594, 66) -> (-116.594, 68)
  line L31 (-116.594, 68) -> (-119.094, 68)
  line L32 (-119.094, 68) -> (-119.094, 68.5)
  line L33 (-119.094, 68.5) -> (-130, 68.5)
  line L34 (-130, 68.5) -> (-130, 68)
  line L35 (-130, 68) -> (-132.5, 68)
  line L36 (-132.5, 68) -> (-132.5, 66)
  line L37 (-132.5, 66) -> (-134.5, 66)
  line L38 (-134.5, 66) -> (-134.5, 63.5)
  line L39 (-134.5, 63.5) -> (-135, 63.5)
  line L40 (-135, 63.5) -> (-135, 8.5)
  line L41 (-135, 8.5) -> (-134.5, 8.5)
  line L42 (-134.5, 8.5) -> (-134.5, 5.5)
  line L43 (-134.5, 5.5) -> (-132.5, 5.5)
  line L44 (-116.5, 3.5) -> (-116.5, 5.5)
  line L45 (-116.5, 5.5) -> (-114.5, 5.5)
  line L46 (-114.5, 5.5) -> (-114.5, 8)
  line L47 (-114.5, 8) -> (-114, 8)
  line L48 (-114, 8) -> (-114, 3)
  line L49 (-114, 3) -> (-119, 3)
  line L50 (-119, 3) -> (-119, 3.5)
  line L51 (-119, 3.5) -> (-116.5, 3.5)
  circle A0 centre (-9.9603, 7.5483) radius 1.25
  circle A1 centre (-111.4603, 7.5483) radius 1.25
  circle A2 centre (-9.9603, 64.0483) radius 1.25
  circle A3 centre (-111.4603, 64.0483) radius 1.25
  line L52 (10.5, 4.5) -> (10.5, 9)
  line L53 (10.5, 9) -> (11, 9)
  line L54 (11, 9) -> (11, 4)
  line L55 (11, 4) -> (6, 4)
  line L56 (6, 4) -> (6, 4.5)
  line L57 (6, 4.5) -> (10.5, 4.5)
  line L58 (-6, 38.5) -> (-5.5, 38.5)
  line L59 (-5.5, 38.5) -> (-5.5, 34)
  line L60 (-5.5, 34) -> (-6, 34)
  line L61 (-6, 34) -> (-6, 38.5)
  dimension "d124" = 0.5
  dimension "d125" = 4.5
  constraint horizontal L58
  constraint vertical L59
  constraint horizontal L60
  constraint vertical L61
  constraint coincident L0.start L3.end
  measures "d124" distance of L0.start L58.end
  measures "d125" distance of L0.start L60.end
extrude "Extrusion29" add sketch "Skizze29" along normal blind 3 contours L3 L58 L59 L60 L61 bodies 1
sketch "Skizze30" plane through (0, 1, 0) normal (0, 1, 0) x (-1, 0, 0)
  line L0 (10.5, 4.5) -> (10.5, 9)
  line L1 (10.5, 9) -> (11, 9)
  line L2 (11, 9) -> (11, 4)
  line L3 (11, 4) -> (6, 4)
  line L4 (6, 4) -> (6, 4.5)
  line L5 (6, 4.5) -> (10.5, 4.5)
  circle A0 centre (-111.4603, 64.0483) radius 1.25
  circle A1 centre (-9.9603, 64.0483) radius 1.25
  circle A2 centre (-111.4603, 7.5483) radius 1.25
  circle A3 centre (-9.9603, 7.5483) radius 1.25
  line L6 (-116.5, 3.5) -> (-116.5, 5.5)
  line L7 (-116.5, 5.5) -> (-114.5, 5.5)
  line L8 (-114.5, 5.5) -> (-114.5, 8)
  line L9 (-114.5, 8) -> (-114, 8)
  line L10 (-114, 8) -> (-114, 3)
  line L11 (-114, 3) -> (-119, 3)
  line L12 (-119, 3) -> (-119, 3.5)
  line L13 (-119, 3.5) -> (-116.5, 3.5)
  line L14 (-132.5, 5.5) -> (-132.5, 3.5)
  line L15 (-132.5, 3.5) -> (-130, 3.5)
  line L16 (-130, 3.5) -> (-130, 3)
  line L17 (-130, 3) -> (-135, 3)
  line L18 (-135, 3) -> (-135, 0)
  line L19 (-135, 0) -> (17, 0)
  line L20 (17, 0) -> (17, 40)
  line L21 (17, 40) -> (0, 40)
  line L22 (0, 40) -> (0, 68.5)
  line L23 (0, 68.5) -> (-114.094, 68.5)
  line L24 (-114.094, 68.5) -> (-114.094, 63.5)
  line L25 (-114.094, 63.5) -> (-114.594, 63.5)
  line L26 (-114.594, 63.5) -> (-114.594, 66)
  line L27 (-114.594, 66) -> (-116.594, 66)
  line L28 (-116.594, 66) -> (-116.594, 68)
  line L29 (-116.594, 68) -> (-119.094, 68)
  line L30 (-119.094, 68) -> (-119.094, 68.5)
  line L31 (-119.094, 68.5) -> (-130, 68.5)
  line L32 (-130, 68.5) -> (-130, 68)
  line L33 (-130, 68) -> (-132.5, 68)
  line L34 (-132.5, 68) -> (-132.5, 66)
  line L35 (-132.5, 66) -> (-134.5, 66)
  line L36 (-134.5, 66) -> (-134.5, 63.5)
  line L37 (-134.5, 63.5) -> (-135, 63.5)
  line L38 (-135, 63.5) -> (-135, 8.5)
  line L39 (-135, 8.5) -> (-134.5, 8.5)
  line L40 (-134.5, 8.5) -> (-134.5, 5.5)
  line L41 (-134.5, 5.5) -> (-132.5, 5.5)
  line L42 (-5.5, 8.9372) -> (-5.5, 4.5)
  line L43 (-5.5, 4.5) -> (-1, 4.5)
  line L44 (-1, 4.5) -> (-1, 4)
  line L45 (-1, 4) -> (-6, 4)
  line L46 (-6, 4) -> (-6, 8.9372)
  line L47 (-6, 8.9372) -> (-5.5, 8.9372)
  line L48 (10.5, 34) -> (10.5, 38.5)
  line L49 (10.5, 38.5) -> (6, 38.5)
  line L50 (6, 38.5) -> (6, 39)
  line L51 (6, 39) -> (11, 39)
  line L52 (11, 39) -> (11, 34)
  line L53 (11, 34) -> (10.5, 34)
  line L54 (-5.5, 38.5) -> (-5.5, 34)
  line L55 (-5.5, 34) -> (-6, 34)
  line L56 (-6, 34) -> (-6, 39)
  line L57 (-6, 39) -> (-1, 39)
  line L58 (-1, 39) -> (-1, 38.5)
  line L59 (-1, 38.5) -> (-5.5, 38.5)
  line L60 (-5.5, 38.5) -> (-3.5, 38.5)
  line L61 (-3.5, 38.5) -> (-3.5, 36.5)
  line L62 (-3.5, 36.5) -> (-5.5, 36.5)
  line L63 (-5.5, 36.5) -> (-5.5, 38.5)
  dimension "d128" = 2
  dimension "d129" = 2
  constraint horizontal L60
  constraint vertical L61
  constraint horizontal L62
  constraint vertical L63
  constraint coincident L54.start L59.end
  measures "d128" distance of L54.start L60.end
  measures "d129" distance of L54.start L62.end